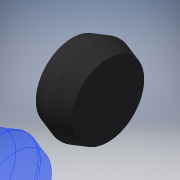
# Autodesk Inventor part: Part_Rubber
Saved by Autodesk Inventor 2019 (Build 230136000, 136)
## iProperties
Created: 2019-04-26
Part Number: Part_Rubber
Material: 고무
Document SubType Name: Modeling
Designer: hinmo
Mass: 115.772 g
Surface Area: 140.621 cm^2
Volume: 124.486 cm^3
Density: 0.93 g/cm^3
Appearance: 고무 - 검은색
Author: hinmo
Autodesk Inventor part; units mm, degrees
ref_plane "YZ Plane" through (0, 0, 0) normal (1, 0, 0) x (0, 1, 0)
ref_plane "XZ Plane" through (0, 0, 0) normal (0, 1, 0) x (-1, 0, 0)
ref_plane "XY Plane" through (0, 0, 0) normal (0, 0, 1) x (1, 0, 0)
sketch "스케치1" plane through (0, 0, 0) normal (1, 0, 0) x (0, 1, 0)
  circle A0 centre (0, 0) radius 37.5
  dimension "d0" = 75
  constraints: 1 centre point, 1 coincident
  measures "d0" diameter of A0
extrude "돌출1" add sketch "스케치1" along normal blind 32
chamfer "모따기1" distance 5 distance2 15 1 edges at (32, -37.5, 0) measured on face at (32, 9.7729, -7.7936)
chamfer "모따기2" distance 5 distance2 15 1 edges at (0, -37.5, 0) measured on face at (0, 9.7729, -7.7936)
sketch "스케치2" plane through (32, 0, 0) normal (1, 0, 0) x (0, 0, -1)
  circle A0 centre (0, 0) radius 6
  dimension "d9" = 12
  constraints: 1 centre point, 1 coincident
  measures "d9" diameter of A0
extrude "돌출2" cut sketch "스케치2" against normal blind 32
